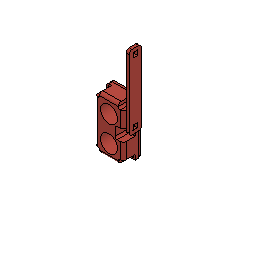
Ultrasonic Sensor Vertical Mount (Autodesk Fusion 360 design; units mm, degrees)
Autodesk Fusion 360 part; units mm, degrees
sketch "Sketch6" plane through (0, 0, -1.722) normal (0, 0, -1) x (-1, 0, 0)
  line L0 (10.914, 23.36) -> (10.914, -23.36)
  line L1 (10.914, -23.36) -> (-10.914, -23.36)
  line L2 (-10.914, -23.36) -> (-10.914, 23.36)
  line L3 (-10.914, 23.36) -> (10.914, 23.36)
  circle A0 centre (-11.914, -24.36) radius 1
  circle A1 centre (-11.914, 24.36) radius 1
  circle A2 centre (11.914, -24.36) radius 1
  circle A3 centre (11.914, 24.36) radius 1
  line L4 (-17.414, -34.5) -> (-14.414, -34.5)
  line L5 (-14.414, -34.5) -> (-14.414, -24.86)
  arc A4 (-14.414, -24.86) -> (-12.414, -26.86) centre (-12.414, -24.86) ccw
  line L6 (-12.414, -26.86) -> (12.414, -26.86)
  arc A5 (12.414, -26.86) -> (14.414, -24.86) centre (12.414, -24.86) ccw
  line L7 (14.414, -24.86) -> (14.414, 24.86)
  arc A6 (14.414, 24.86) -> (12.414, 26.86) centre (12.414, 24.86) ccw
  line L8 (12.414, 26.86) -> (-12.414, 26.86)
  arc A7 (-12.414, 26.86) -> (-14.414, 24.86) centre (-12.414, 24.86) ccw
  line L9 (-14.414, 24.86) -> (-14.414, 34.5)
  line L10 (-14.414, 34.5) -> (-17.414, 34.5)
  line L11 (-17.414, 34.5) -> (-17.414, -34.5)
  line L12 (-12.414, 26.86) -> (-14.414, 26.86)
  line L13 (-12.414, -26.86) -> (-14.414, -26.86)
sketch "Sketch7" plane through (14.414, 0, 0) normal (1, 0, 0) x (0, 0, -1)
  line L0 (-10.97, 21.86) -> (-10.97, 5.83)
  line L1 (-10.97, 5.83) -> (-1.778, 5.83)
  line L2 (-1.778, 5.83) -> (-1.778, -5.83)
  line L3 (-1.778, -5.83) -> (-10.97, -5.83)
  line L4 (-10.97, -5.83) -> (-10.97, -21.86)
  line L5 (-10.97, -21.86) -> (-1.97, -21.86)
  line L6 (-1.97, -21.86) -> (-1.97, -24.86)
  line L7 (-1.97, -24.86) -> (1.722, -24.86)
  line L8 (1.722, -24.86) -> (1.722, 24.86)
  line L9 (1.722, 24.86) -> (-1.97, 24.86)
  line L10 (-1.97, 24.86) -> (-1.97, 21.86)
  line L11 (-1.97, 21.86) -> (-10.97, 21.86)
  line L12 (-13.97, -3.83) -> (-13.97, 3.83)
  line L13 (3.722, 24.86) -> (3.722, -24.86)
  line L14 (-4.62, 69.25) -> (-17.32, 69.25) construction
  line L15 (-17.32, 69.25) -> (-17.32, 5.75) construction
  line L16 (-17.32, 5.75) -> (-4.62, 5.75) construction
  line L17 (-4.62, 5.75) -> (-4.62, 69.25) construction
  line L18 (-4.62, 69.25) -> (-17.32, 5.75) construction
  line L19 (-17.32, 69.25) -> (-4.62, 5.75) construction
  line L20 (3.722, 0) -> (-13.97, 0) construction
  line L21 (-2.27, 66.9) -> (-6.97, 66.9)
  line L22 (-6.97, 66.9) -> (-6.97, 71.6)
  line L23 (-6.97, 71.6) -> (-2.27, 71.6)
  line L24 (-2.27, 71.6) -> (-2.27, 66.9)
  line L25 (-2.27, 66.9) -> (-6.97, 71.6) construction
  line L26 (-6.97, 66.9) -> (-2.27, 71.6) construction
  line L27 (-19.67, 71.6) -> (-14.97, 71.6)
  line L28 (-14.97, 71.6) -> (-14.97, 66.9)
  line L29 (-14.97, 66.9) -> (-19.67, 66.9)
  line L30 (-19.67, 66.9) -> (-19.67, 71.6)
  line L31 (-6.97, 8.1) -> (-2.27, 8.1)
  line L32 (-2.27, 8.1) -> (-2.27, 3.4)
  line L33 (-2.27, 3.4) -> (-6.97, 3.4)
  line L34 (-6.97, 3.4) -> (-6.97, 8.1)
  line L35 (-19.67, 8.1) -> (-14.97, 8.1)
  line L36 (-14.97, 8.1) -> (-14.97, 3.4)
  line L37 (-14.97, 3.4) -> (-19.67, 3.4)
  line L38 (-19.67, 3.4) -> (-19.67, 8.1)
  line L39 (1.722, 0) -> (-23.662, 0)
  line L40 (-23.662, 0) -> (-23.662, 75)
  line L41 (-23.662, 75) -> (1.722, 75)
  line L42 (1.722, 75) -> (1.722, 0)
  line L43 (1.722, 0) -> (-23.662, 75) construction
  line L44 (-23.662, 0) -> (1.722, 75) construction
  line L45 (-10.97, 75) -> (-10.97, 0)
  dimension "d1" = 12.7
  dimension "d2" = 63.5
  dimension "d3" = 4.7
  dimension "d4" = 75
  dimension "d5" = 0
  measures "d5" distance of L20
sketch "Sketch8" plane through (0, 0, -3.722) normal (0, 0, -1) x (-1, 0, 0)
  arc A0 (-15.5, 37.5) -> (-17.5, 35.5) centre (-15.5, 35.5) ccw
  line L0 (-17.5, 35.5) -> (-17.5, -35.5)
  arc A1 (-17.5, -35.5) -> (-15.5, -37.5) centre (-15.5, -35.5) ccw
  line L1 (-15.5, -37.5) -> (15.5, -37.5)
  arc A2 (15.5, -37.5) -> (17.5, -35.5) centre (15.5, -35.5) ccw
  line L2 (17.5, -35.5) -> (17.5, 35.5)
  arc A3 (17.5, 35.5) -> (15.5, 37.5) centre (15.5, 35.5) ccw
  line L3 (15.5, 37.5) -> (-15.5, 37.5)
  circle A4 centre (-11.914, -24.36) radius 1
  line L4 (-8.2883, -5.83) -> (-10.914, -5.83)
  line L5 (-10.914, -5.83) -> (-10.914, 5.83)
  line L6 (-10.914, 5.83) -> (-8.2883, 5.83)
  arc A5 (-6.2883, 3.83) -> (-8.2883, 5.83) centre (-8.2883, 3.83) ccw
  line L7 (-6.2883, 3.83) -> (-6.2883, -3.83)
  arc A6 (-8.2883, -5.83) -> (-6.2883, -3.83) centre (-8.2883, -3.83) ccw
  line L8 (-10.414, 29.464) -> (-14.986, 29.464)
  line L9 (-14.986, 29.464) -> (-14.986, 34.036)
  line L10 (-14.986, 34.036) -> (-10.414, 34.036)
  line L11 (-10.414, 34.036) -> (-10.414, 29.464)
  line L12 (14.986, 29.464) -> (10.414, 29.464)
  line L13 (10.414, 29.464) -> (10.414, 34.036)
  line L14 (10.414, 34.036) -> (14.986, 34.036)
  line L15 (14.986, 34.036) -> (14.986, 29.464)
  circle A7 centre (11.914, 24.36) radius 1
  circle A8 centre (-11.914, 24.36) radius 1
  circle A9 centre (11.914, -24.36) radius 1
  line L16 (10.414, -34.036) -> (10.414, -29.464)
  line L17 (10.414, -29.464) -> (14.986, -29.464)
  line L18 (14.986, -29.464) -> (14.986, -34.036)
  line L19 (14.986, -34.036) -> (10.414, -34.036)
  line L20 (-14.986, -34.036) -> (-14.986, -29.464)
  line L21 (-14.986, -29.464) -> (-10.414, -29.464)
  line L22 (-10.414, -29.464) -> (-10.414, -34.036)
  line L23 (-10.414, -34.036) -> (-14.986, -34.036)
  line L24 (12.414, 26.86) -> (-12.414, 26.86)
  arc A10 (14.414, 24.86) -> (12.414, 26.86) centre (12.414, 24.86) ccw
  line L25 (14.414, -24.86) -> (14.414, 24.86)
  arc A11 (12.414, -26.86) -> (14.414, -24.86) centre (12.414, -24.86) ccw
  line L26 (-12.414, -26.86) -> (12.414, -26.86)
  arc A12 (-14.414, -24.86) -> (-12.414, -26.86) centre (-12.414, -24.86) ccw
  line L27 (-14.414, 24.86) -> (-14.414, -24.86)
  arc A13 (-12.414, 26.86) -> (-14.414, 24.86) centre (-12.414, 24.86) ccw
  arc A14 (-15.5, 37.5) -> (-17.5, 35.5) centre (-15.5, 35.5) ccw
  line L28 (-15.5, 37.5) -> (15.5, 37.5)
  arc A15 (17.5, 35.5) -> (15.5, 37.5) centre (15.5, 35.5) ccw
  line L29 (17.5, 35.5) -> (17.5, -35.5)
  arc A16 (15.5, -37.5) -> (17.5, -35.5) centre (15.5, -35.5) ccw
  line L30 (15.5, -37.5) -> (-15.5, -37.5)
  arc A17 (-17.5, -35.5) -> (-15.5, -37.5) centre (-15.5, -35.5) ccw
  line L31 (-17.5, -35.5) -> (-17.5, 35.5)
  line L32 (-14.986, -29.464) -> (-14.986, -34.036)
  line L33 (-14.986, -34.036) -> (-10.414, -34.036)
  line L34 (-10.414, -34.036) -> (-10.414, -29.464)
  line L35 (-10.414, -29.464) -> (-14.986, -29.464)
  line L36 (10.414, -29.464) -> (10.414, -34.036)
  line L37 (10.414, -34.036) -> (14.986, -34.036)
  line L38 (14.986, -34.036) -> (14.986, -29.464)
  line L39 (14.986, -29.464) -> (10.414, -29.464)
  circle A18 centre (11.914, -24.36) radius 1
  circle A19 centre (-11.914, 24.36) radius 1
  circle A20 centre (11.914, 24.36) radius 1
  line L40 (10.414, 29.464) -> (14.986, 29.464)
  line L41 (14.986, 29.464) -> (14.986, 34.036)
  line L42 (14.986, 34.036) -> (10.414, 34.036)
  line L43 (10.414, 34.036) -> (10.414, 29.464)
  line L44 (-14.986, 29.464) -> (-10.414, 29.464)
  line L45 (-10.414, 29.464) -> (-10.414, 34.036)
  line L46 (-10.414, 34.036) -> (-14.986, 34.036)
  line L47 (-14.986, 34.036) -> (-14.986, 29.464)
  line L48 (-10.914, 23.36) -> (-10.914, -23.36)
  line L49 (-10.914, -23.36) -> (10.914, -23.36)
  line L50 (10.914, -23.36) -> (10.914, 23.36)
  line L51 (10.914, 23.36) -> (-10.914, 23.36)
  circle A21 centre (-11.914, -24.36) radius 1
sketch "Sketch1" plane through (0, 0, 1.778) normal (0, 0, 1) x (1, 0, 0)
  line L0 (10.414, -22.86) -> (10.414, 22.86)
  line L1 (10.414, 22.86) -> (-10.414, 22.86)
  line L2 (-10.414, 22.86) -> (-10.414, -22.86)
  line L3 (-10.414, -22.86) -> (10.414, -22.86)
  circle A0 centre (8.3312, -20.7772) radius 1.0668
  circle A1 centre (-8.3312, 20.7772) radius 1.0668
  line L4 (10.414, -22.86) -> (10.414, 22.86)
  line L5 (-10.414, -22.86) -> (10.414, -22.86)
  line L6 (-10.414, 22.86) -> (-10.414, -22.86)
  line L7 (10.414, 22.86) -> (-10.414, 22.86)
  circle A2 centre (0, 12.5374) radius 8.067
  circle A3 centre (0, -13.3706) radius 8.067
  line L8 (-10.914, 23.36) -> (-10.914, -23.36)
  line L9 (-10.914, -23.36) -> (10.914, -23.36)
  line L10 (10.914, -23.36) -> (10.914, 23.36)
  line L11 (10.914, 23.36) -> (-10.914, 23.36)
  circle A4 centre (0, -13.3706) radius 8.567
  circle A5 centre (0, 12.5374) radius 8.567
  line L12 (7.0383, 5.08) -> (7.0383, -5.08)
  line L13 (7.0383, -5.08) -> (10.0863, -5.08)
  line L14 (10.0863, -5.08) -> (10.0863, 5.08)
  line L15 (10.0863, 5.08) -> (7.0383, 5.08)
  line L16 (6.2883, 5.83) -> (6.2883, -5.83)
  line L17 (6.2883, -5.83) -> (10.8363, -5.83)
  line L18 (10.8363, -5.83) -> (10.8363, 5.83)
  line L19 (10.8363, 5.83) -> (6.2883, 5.83)
  line L20 (-14.414, 26.86) -> (-14.414, -26.86)
  line L21 (-14.414, -26.86) -> (14.414, -26.86)
  line L22 (14.414, -26.86) -> (14.414, 26.86)
  line L23 (14.414, 26.86) -> (-14.414, 26.86)
  line L24 (-5.914, 6) -> (-10.914, 6)
  line L25 (-10.914, 6) -> (-10.914, -6)
  line L26 (-10.914, -6) -> (-5.914, -6)
  line L27 (-5.914, -6) -> (-5.914, 6)
  line L28 (10.8363, 5.83) -> (14.414, 5.83)
  line L29 (14.414, 5.83) -> (14.414, -5.83)
  line L30 (14.414, -5.83) -> (10.8363, -5.83)
  line L31 (10.8363, -5.83) -> (10.8363, 5.83)
  dimension "d1_1" = 0.5
  dimension "d2_1" = 0.5
  dimension "d3_1" = 0.5
  dimension "d4_1" = 0.75
  dimension "d5_1" = 4
  dimension "d12_1" = 5
  dimension "d13_1" = 6
  dimension "d14_1" = 6
  measures "d1_1" distance of L2
  measures "d4_1" distance of L12
  measures "d5_1" distance of L2
  measures "d13_1" distance of origin
  measures "d14_1" distance of origin
extrude "Extrude1" add sketch "Sketch1" along normal blind 12.192 contours L0 L1 L2 L3 L4 L5 L6 L7 L16 L17 L19 L24 L26 L27 | L0 L2 L3 L4 L5 L6 L8 L9 L10 L17 L26 L30 | L0 L1 L2 L4 L6 L7 L8 L10 L11 L19 L24 L28 | L2 L6 L8 L24 L25 L26 | L2 L6 L24 L26 L27 | L8 L9 L10 L11 L20 L21 L22 L23 L25 L28 L30 | A0 | A1 makes body 1
fillet "Fillet1" radius 2 2 edges at (6.2883, 5.83, 7.874) (6.2883, -5.83, 7.874) on bodies 1
extrude "Extrude2" cut sketch "Sketch1" along normal blind 5 contours L2 L6 L8 L24 L25 L26 | L2 L6 L24 L26 L27 bodies 1
fillet "Fillet2" radius 2 2 edges at (-5.914, -6, 4.278) (-5.914, 6, 4.278) on bodies 1
extrude "Extrude3" add sketch "Sketch1" against normal blind 3.5 contours L8 L9 L10 L11 L20 L21 L22 L23 L25 L28 L30 | L10 L22 L28 L29 L30 bodies 1
sketch "Sketch2" plane through (0, 0, -1.722) normal (0, 0, -1) x (-1, 0, 0)
  line L0 (10.914, 23.36) -> (10.914, -23.36)
  line L1 (10.914, -23.36) -> (-10.914, -23.36)
  line L2 (-10.914, -23.36) -> (-10.914, 23.36)
  line L3 (-10.914, 23.36) -> (10.914, 23.36)
  line L4 (14.414, 26.86) -> (-14.414, 26.86)
  line L5 (-14.414, 26.86) -> (-14.414, -26.86)
  line L6 (-14.414, -26.86) -> (14.414, -26.86)
  line L7 (14.414, -26.86) -> (14.414, 26.86)
  circle A0 centre (-11.914, 24.36) radius 1
  circle A1 centre (11.914, 24.36) radius 1
  circle A2 centre (11.914, -24.36) radius 1
  circle A3 centre (-11.914, -24.36) radius 1
  line L8 (-14.414, -26.86) -> (-14.414, 26.86)
  line L9 (14.414, -26.86) -> (-14.414, -26.86)
  line L10 (14.414, 26.86) -> (14.414, -26.86)
  dimension "d18_1" = 2
  dimension "d19_1" = 2.5
  dimension "d20_1" = 2.5
  dimension "d21_1" = 2.5
  dimension "d22_1" = 2.5
  measures "d18_1" diameter of A3
  measures "d19_1" distance of L8
  measures "d20_1" distance of L9
  measures "d21_1" distance of L4
  measures "d22_1" distance of L10
extrude "Extrude4" cut sketch "Sketch2" against normal blind 15.692 contours A0 | A1 | A2 | A3 bodies 1
sketch "Sketch3" plane through (0, 0, 13.97) normal (0, 0, 1) x (1, 0, 0)
  circle A0 centre (-11.914, 24.36) radius 1
  circle A1 centre (-11.914, -24.36) radius 1
  circle A2 centre (11.914, 24.36) radius 1
  circle A3 centre (11.914, -24.36) radius 1
  circle A4 centre (0, -13.3706) radius 8.567
  circle A5 centre (0, 12.5374) radius 8.567
  line L0 (8.2883, 5.83) -> (14.414, 5.83)
  line L1 (14.414, 5.83) -> (14.414, 26.86)
  line L2 (14.414, 26.86) -> (-14.414, 26.86)
  line L3 (-14.414, 26.86) -> (-14.414, -26.86)
  line L4 (-14.414, -26.86) -> (14.414, -26.86)
  line L5 (14.414, -26.86) -> (14.414, -5.83)
  line L6 (14.414, -5.83) -> (8.2883, -5.83)
  arc A6 (6.2883, -3.83) -> (8.2883, -5.83) centre (8.2883, -3.83) ccw
  line L7 (6.2883, -3.83) -> (6.2883, 3.83)
  arc A7 (8.2883, 5.83) -> (6.2883, 3.83) centre (8.2883, 3.83) ccw
  circle A8 centre (-11.914, -24.36) radius 1
  circle A9 centre (11.914, -24.36) radius 1
  circle A10 centre (11.914, 24.36) radius 1
  circle A11 centre (-11.914, 24.36) radius 1
  line L8 (-14.414, 26.86) -> (-9.414, 26.86)
  line L9 (-9.414, 26.86) -> (-9.414, 21.86)
  line L10 (-9.414, 21.86) -> (-14.414, 21.86)
  line L11 (-14.414, 21.86) -> (-14.414, 26.86)
  line L12 (-14.414, 26.86) -> (-9.414, 21.86) construction
  line L13 (-9.414, 26.86) -> (-14.414, 21.86) construction
  line L14 (14.414, 26.86) -> (9.414, 26.86)
  line L15 (9.414, 26.86) -> (9.414, 21.86)
  line L16 (9.414, 21.86) -> (14.414, 21.86)
  line L17 (14.414, 21.86) -> (14.414, 26.86)
  line L18 (14.414, 26.86) -> (9.414, 21.86) construction
  line L19 (9.414, 26.86) -> (14.414, 21.86) construction
  line L20 (14.414, -26.86) -> (9.414, -26.86)
  line L21 (9.414, -26.86) -> (9.414, -21.86)
  line L22 (9.414, -21.86) -> (14.414, -21.86)
  line L23 (14.414, -21.86) -> (14.414, -26.86)
  line L24 (14.414, -26.86) -> (9.414, -21.86) construction
  line L25 (9.414, -26.86) -> (14.414, -21.86) construction
  line L26 (-14.414, -26.86) -> (-9.414, -26.86)
  line L27 (-9.414, -26.86) -> (-9.414, -21.86)
  line L28 (-9.414, -21.86) -> (-14.414, -21.86)
  line L29 (-14.414, -21.86) -> (-14.414, -26.86)
  line L30 (-14.414, -26.86) -> (-9.414, -21.86) construction
  line L31 (-9.414, -26.86) -> (-14.414, -21.86) construction
extrude "Extrude5" cut sketch "Sketch3" against normal blind 12 contours L1 L2 L14 L15 L16 L17 | L2 L3 L8 L9 L10 L11 | L4 L5 L20 L21 L22 L23 | L3 L4 L26 L27 L28 L29 bodies 1
fillet "Fillet3" radius 2 8 edges at (-9.414, 21.86, 7.97) (9.414, 21.86, 7.97) (9.414, -21.86, 7.97) (-9.414, -21.86, 7.97) (14.414, -26.86, 0.124) (14.414, 26.86, 0.124) (-14.414, 26.86, 0.124) (-14.414, -26.86, 0.124) on bodies 1
sketch "Sketch4" plane through (0, 0, -1.722) normal (0, 0, -1) x (-1, 0, 0)
  arc A0 (12.414, -26.86) -> (14.414, -24.86) centre (12.414, -24.86) ccw
  line L0 (14.414, -24.86) -> (14.414, 24.86)
  arc A1 (14.414, 24.86) -> (12.414, 26.86) centre (12.414, 24.86) ccw
  line L1 (12.414, 26.86) -> (-12.414, 26.86)
  arc A2 (-12.414, 26.86) -> (-14.414, 24.86) centre (-12.414, 24.86) ccw
  line L2 (-14.414, 24.86) -> (-14.414, -24.86)
  arc A3 (-14.414, -24.86) -> (-12.414, -26.86) centre (-12.414, -24.86) ccw
  line L3 (-12.414, -26.86) -> (12.414, -26.86)
  circle A4 centre (11.914, 24.36) radius 1
  circle A5 centre (11.914, -24.36) radius 1
  circle A6 centre (-11.914, 24.36) radius 1
  circle A7 centre (-11.914, -24.36) radius 1
  line L4 (10.914, 23.36) -> (10.914, -23.36)
  line L5 (10.914, -23.36) -> (-10.914, -23.36)
  line L6 (-10.914, -23.36) -> (-10.914, 23.36)
  line L7 (-10.914, 23.36) -> (10.914, 23.36)
  line L8 (-14.414, 0) -> (15, 0) construction
  line L9 (-12.7, -31.75) -> (12.7, -31.75)
  line L10 (12.7, -31.75) -> (12.7, 31.75)
  line L11 (12.7, 31.75) -> (-12.7, 31.75)
  line L12 (-12.7, 31.75) -> (-12.7, -31.75)
  line L13 (-12.7, -31.75) -> (12.7, 31.75) construction
  line L14 (12.7, -31.75) -> (-12.7, 31.75) construction
  line L15 (-14.986, -34.036) -> (-10.414, -34.036)
  line L16 (-10.414, -34.036) -> (-10.414, -29.464)
  line L17 (-10.414, -29.464) -> (-14.986, -29.464)
  line L18 (-14.986, -29.464) -> (-14.986, -34.036)
  line L19 (-14.986, -34.036) -> (-10.414, -29.464) construction
  line L20 (-10.414, -34.036) -> (-14.986, -29.464) construction
  line L21 (10.414, -34.036) -> (14.986, -34.036)
  line L22 (14.986, -34.036) -> (14.986, -29.464)
  line L23 (14.986, -29.464) -> (10.414, -29.464)
  line L24 (10.414, -29.464) -> (10.414, -34.036)
  line L25 (10.414, -34.036) -> (14.986, -29.464) construction
  line L26 (14.986, -34.036) -> (10.414, -29.464) construction
  line L27 (10.414, 34.036) -> (14.986, 34.036)
  line L28 (14.986, 34.036) -> (14.986, 29.464)
  line L29 (14.986, 29.464) -> (10.414, 29.464)
  line L30 (10.414, 29.464) -> (10.414, 34.036)
  line L31 (10.414, 34.036) -> (14.986, 29.464) construction
  line L32 (14.986, 34.036) -> (10.414, 29.464) construction
  line L33 (-14.986, 34.036) -> (-10.414, 34.036)
  line L34 (-10.414, 34.036) -> (-10.414, 29.464)
  line L35 (-10.414, 29.464) -> (-14.986, 29.464)
  line L36 (-14.986, 29.464) -> (-14.986, 34.036)
  line L37 (-14.986, 34.036) -> (-10.414, 29.464) construction
  line L38 (-10.414, 34.036) -> (-14.986, 29.464) construction
  line L39 (-17.5, -37.5) -> (17.5, -37.5)
  line L40 (17.5, -37.5) -> (17.5, 37.5)
  line L41 (17.5, 37.5) -> (-17.5, 37.5)
  line L42 (-17.5, 37.5) -> (-17.5, -37.5)
  line L43 (-17.5, -37.5) -> (17.5, 37.5) construction
  line L44 (17.5, -37.5) -> (-17.5, 37.5) construction
  line L45 (-14.414, -5.83) -> (-8.2883, -5.83)
  arc A8 (-8.2883, -5.83) -> (-6.2883, -3.83) centre (-8.2883, -3.83) ccw
  line L46 (-6.2883, -3.83) -> (-6.2883, 3.83)
  arc A9 (-6.2883, 3.83) -> (-8.2883, 5.83) centre (-8.2883, 3.83) ccw
  line L47 (-8.2883, 5.83) -> (-14.414, 5.83)
  line L48 (-10.914, -23.36) -> (-10.914, 23.36)
  dimension "d28_1" = 63.5
  dimension "d29_1" = 25.4
  dimension "d30_1" = 4.572
  dimension "d31_1" = 35
  dimension "d32_1" = 75
extrude "Extrude6" add sketch "Sketch4" along normal blind 2 separate body contours A0 A1 L1 A2 A3 L3 A4 A5 A6 A7 L4 L5 L6 L7 L10 L12 L45 L47 L48 | A0 A3 L3 L9 L10 L12 L16 L17 L23 L24 | A0 L0 A1 A4 A5 L10 | L2 A3 A7 L12 L45 | A1 L1 A2 L10 L11 L12 L29 L30 L34 L35 | L2 L12 L45 L47 | A2 L2 A6 L12 L47 | L6 L12 L45 L47 L48 | L4 L5 L6 L7 L45 A8 L46 A9 L47 L48 | L39 L40 L41 L42 makes body 2
fillet "Fillet4" radius 2 4 edges at (17.5, -37.5, -2.722) (-17.5, -37.5, -2.722) (-17.5, 37.5, -2.722) (17.5, 37.5, -2.722) on bodies 2
fillet "Fillet5" radius 3 5 edges at (14.414, -13.845, 13.97) (0, -26.86, 13.97) (-14.414, 0, 13.97) (14.414, 13.845, 13.97) (0, 26.86, 13.97) on bodies 1
sketch "Sketch5" plane through (0, 0, -1.722) normal (0, 0, 1) x (1, 0, 0)
  line L0 (14.986, 29.464) -> (10.414, 29.464)
  line L1 (10.414, 29.464) -> (10.414, 34.036)
  line L2 (10.414, 34.036) -> (14.986, 34.036)
  line L3 (14.986, 34.036) -> (14.986, 29.464)
  circle A0 centre (11.914, -24.36) radius 1
  line L4 (14.986, -29.464) -> (14.986, -34.036)
  line L5 (14.986, -34.036) -> (10.414, -34.036)
  line L6 (10.414, -34.036) -> (10.414, -29.464)
  line L7 (10.414, -29.464) -> (14.986, -29.464)
  line L8 (-10.414, -29.464) -> (-10.414, -34.036)
  line L9 (-10.414, -34.036) -> (-14.986, -34.036)
  line L10 (-14.986, -34.036) -> (-14.986, -29.464)
  line L11 (-14.986, -29.464) -> (-10.414, -29.464)
  circle A1 centre (11.914, 24.36) radius 1
  line L12 (10.914, -5.83) -> (8.2883, -5.83)
  arc A2 (6.2883, -3.83) -> (8.2883, -5.83) centre (8.2883, -3.83) ccw
  line L13 (6.2883, -3.83) -> (6.2883, 3.83)
  arc A3 (8.2883, 5.83) -> (6.2883, 3.83) centre (8.2883, 3.83) ccw
  line L14 (8.2883, 5.83) -> (10.914, 5.83)
  line L15 (10.914, 5.83) -> (10.914, -5.83)
  line L16 (-10.414, 29.464) -> (-14.986, 29.464)
  line L17 (-14.986, 29.464) -> (-14.986, 34.036)
  line L18 (-14.986, 34.036) -> (-10.414, 34.036)
  line L19 (-10.414, 34.036) -> (-10.414, 29.464)
  circle A4 centre (-11.914, 24.36) radius 1
  circle A5 centre (-11.914, -24.36) radius 1
  arc A6 (17.5, 35.5) -> (15.5, 37.5) centre (15.5, 35.5) ccw
  line L20 (15.5, 37.5) -> (-15.5, 37.5)
  arc A7 (-15.5, 37.5) -> (-17.5, 35.5) centre (-15.5, 35.5) ccw
  line L21 (-17.5, 35.5) -> (-17.5, -35.5)
  arc A8 (-17.5, -35.5) -> (-15.5, -37.5) centre (-15.5, -35.5) ccw
  line L22 (-15.5, -37.5) -> (15.5, -37.5)
  arc A9 (15.5, -37.5) -> (17.5, -35.5) centre (15.5, -35.5) ccw
  line L23 (17.5, -35.5) -> (17.5, 35.5)
  line L24 (-10.914, -23.36) -> (10.914, -23.36)
  line L25 (10.914, -23.36) -> (10.914, 23.36)
  line L26 (-10.914, 23.36) -> (-10.914, -23.36)
  line L27 (10.914, 23.36) -> (-10.914, 23.36)
extrude "Extrude7" cut sketch "Sketch5" against normal blind 1 contours L12 A2 L13 A3 L14 L24 L25 L26 L27 bodies 2
extrude "Extrude8" cut sketch "Sketch8" against normal blind 5.692 contours A0 L0 A1 L1 A2 L2 A3 L3 A14 L28 A15 L29 A16 L30 A17 L31 bodies 2
extrude "Extrude9" add sketch "Sketch7" along normal blind 3 contours L0 L1 L2 L8 L9 L10 L11 L31 L32 L34 L39 L42 L45 | L9 L10 L11 L41 L42 L45 | L1 L2 L32 L33 L34 L39 L45 bodies 1
fillet "Fillet6" radius 3 4 edges at (15.914, 75, -1.722) (15.914, 75, 10.97) (15.914, 0, -1.722) (15.914, 0, 10.97) on bodies 1
extrude "Extrude10" add sketch "Sketch6" against normal blind 3.692 contours L5 A4 L13 | A7 L9 L12 bodies 1
equation "d1 = ( 25.4 / 2 ) * 1 mm"
equation "d2 = ( ( 25.4 / 2 ) * 5 ) * 1 mm"
equation "d5 = d49 / 2"
named bodies: "Ultrasoinc Top 2", "Ultrasonic Bottom 2"
